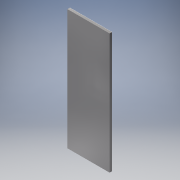
# Autodesk Inventor part: Etichetta
Saved by Autodesk Inventor 2016 (Build 200138000, 138)
## iProperties
Created: 2016-09-10
Part Number: Etichetta
Material: Generic
Document SubType Name: Modeling
Designer: Muhammad
Density: 1 g/cm^3
Appearance: Knurled 45
Author: Muhammad
Autodesk Inventor part; units mm, degrees
(part 1 of 2)
ref_plane "YZ Plane" through (0, 0, 0) normal (1, 0, 0) x (0, 1, 0)
ref_plane "XZ Plane" through (0, 0, 0) normal (0, 1, 0) x (-1, 0, 0)
ref_plane "XY Plane" through (0, 0, 0) normal (0, 0, 1) x (1, 0, 0)
sketch "Sketch1" plane through (0, 0, 0) normal (0, 1, 0) x (-1, 0, 0)
  line L0 (14, 40) -> (-14, 40)
  line L1 (-14, 40) -> (-14, -40)
  line L2 (-14, -40) -> (14, -40)
  line L3 (14, -40) -> (14, 40)
  line L4 (14, 40) -> (-14, -40) construction
  line L5 (-14, 40) -> (14, -40) construction
  point P0 (0, 0)
  dimension "d0" = 28
  dimension "d1" = 80
  constraints: 12 end point, 2 midpoint, 2 parallel, 1 horizontal, 1 perpendicular
  measures "d0" distance of L2.end L1.end
  measures "d1" distance of L1.end L0.end
extrude "Extrusion1" add sketch "Sketch1" along normal blind 2
fillet "Fillet1" radius 0.5 4 edges at (-14, 2, 0) (0, 2, 40) (14, 2, 0) (0, 2, -40)
sketch "Sketch3" plane through (0, 2, 0) normal (0, 1, 0) x (1, 0, 0)
  line L0 (-11.1237, -27.6216) -> (-11.1237, 26.8213) construction
  line L1 (-11.1237, 26.8213) -> (10.7875, 26.8213) construction
  line L2 (10.7875, 26.8213) -> (10.7875, -27.6216) construction
  line L3 (10.7875, -27.6216) -> (-11.1237, -27.6216) construction
  line L4 (-14, 40) -> (-14, -40) construction
  line L5 (-14, 0) -> (0, 0) construction
  spline S0 degree 2 poles (-8.5426, -15.8821) (-8.2817, -15.8821) (-7.8818, -16.0806) (-7.7513, -16.2451) knots 0 0 0 1 2 2 2
  spline S1 degree 2 poles (-7.7513, -16.2451) (-7.5982, -16.4437) (-7.4677, -16.8947) (-7.4677, -17.252) knots 0 0 0 1 2 2 2
  line L6 (-7.4677, -17.252) -> (-7.4677, -18.2561)
  line L7 (-7.4677, -18.2561) -> (-10.9677, -18.2561)
  line L8 (-10.9677, -18.2561) -> (-10.9677, -17.3286)
  spline S2 degree 2 poles (-10.9677, -17.3286) (-10.9677, -16.9542) (-10.9195, -16.5798) (-10.8259, -16.4097) knots 0 0 0 1 2 2 2
  spline S3 degree 2 poles (-10.8259, -16.4097) (-10.7266, -16.2196) (-10.4004, -16.0466) (-10.1792, -16.0466) knots 0 0 0 1 2 2 2
  spline S4 degree 2 poles (-10.1792, -16.0466) (-9.9324, -16.0466) (-9.541, -16.3075) (-9.4304, -16.5373) knots 0 0 0 1 2 2 2
  line L9 (-9.4304, -16.5373) -> (-9.4134, -16.5373)
  spline S5 degree 2 poles (-9.4134, -16.5373) (-9.3283, -16.2253) (-8.8773, -15.8821) (-8.5426, -15.8821) knots 0 0 0 1 2 2 2
  spline S6 degree 2 poles (-8.5228, -16.3671) (-8.7213, -16.3671) (-8.9766, -16.4806) (-9.0674, -16.6507) knots 0 0 0 1 2 2 2
  spline S7 degree 2 poles (-9.0674, -16.6507) (-9.1241, -16.7614) (-9.1581, -17.0223) (-9.1581, -17.2634) knots 0 0 0 1 2 2 2
  line L10 (-9.1581, -17.2634) -> (-9.1581, -17.7909)
  line L11 (-9.1581, -17.7909) -> (-7.8648, -17.7909)
  line L12 (-7.8648, -17.7909) -> (-7.8648, -17.4137)
  spline S8 degree 2 poles (-7.8648, -17.4137) (-7.8648, -17.1074) (-7.9215, -16.7557) (-8.0123, -16.6195) knots 0 0 0 1 2 2 2
  spline S9 degree 2 poles (-8.0123, -16.6195) (-8.1059, -16.4891) (-8.3384, -16.3671) (-8.5228, -16.3671) knots 0 0 0 1 2 2 2
  spline S10 degree 2 poles (-10.114, -16.5316) (-10.2388, -16.5316) (-10.426, -16.6167) (-10.4798, -16.7103) knots 0 0 0 1 2 2 2
  spline S11 degree 2 poles (-10.4798, -16.7103) (-10.5422, -16.8238) (-10.5706, -17.0989) (-10.5706, -17.3456) knots 0 0 0 1 2 2 2
  line L13 (-10.5706, -17.3456) -> (-10.5706, -17.7909)
  line L14 (-10.5706, -17.7909) -> (-9.5467, -17.7909)
  line L15 (-9.5467, -17.7909) -> (-9.5467, -17.2634)
  spline S12 degree 2 poles (-9.5467, -17.2634) (-9.5467, -17.045) (-9.5921, -16.8379) (-9.663, -16.7273) knots 0 0 0 1 2 2 2
  spline S13 degree 2 poles (-9.663, -16.7273) (-9.7311, -16.6195) (-9.9495, -16.5316) (-10.114, -16.5316) knots 0 0 0 1 2 2 2
  spline S14 degree 2 poles (-7.4081, -14.3136) (-7.4081, -14.9433) (-8.1144, -15.6353) (-8.7667, -15.6353) knots 0 0 0 1 2 2 2
  spline S15 degree 2 poles (-8.7667, -15.6353) (-9.4077, -15.6353) (-10.1678, -14.9631) (-10.1678, -14.4214) knots 0 0 0 1 2 2 2
  spline S16 degree 2 poles (-10.1678, -14.4214) (-10.1678, -14.1775) (-10.026, -13.8003) (-9.8757, -13.6613) knots 0 0 0 1 2 2 2
  spline S17 degree 2 poles (-9.8757, -13.6613) (-9.7254, -13.5195) (-9.2914, -13.3691) (-8.9766, -13.3691) knots 0 0 0 1 2 2 2
  line L16 (-8.9766, -13.3691) -> (-8.7355, -13.3691)
  line L17 (-8.7355, -13.3691) -> (-8.7355, -15.1872)
  spline S18 degree 2 poles (-8.7355, -15.1872) (-8.2789, -15.1872) (-7.7939, -14.7277) (-7.7939, -14.3193) knots 0 0 0 1 2 2 2
  spline S19 degree 2 poles (-7.7939, -14.3193) (-7.7939, -14.1746) (-7.8591, -13.8939) (-7.9102, -13.7804) knots 0 0 0 1 2 2 2
  spline S20 degree 2 poles (-7.9102, -13.7804) (-7.9669, -13.6613) (-8.0661, -13.4968) (-8.1115, -13.4429) knots 0 0 0 1 2 2 2
  line L18 (-8.1115, -13.4429) -> (-8.1115, -13.4174)
  line L19 (-8.1115, -13.4174) -> (-7.6294, -13.4174)
  spline S21 degree 2 poles (-7.6294, -13.4174) (-7.5982, -13.4939) (-7.5074, -13.7265) (-7.4819, -13.8173) knots 0 0 0 1 2 2 2
  spline S22 degree 2 poles (-7.4819, -13.8173) (-7.445, -13.9449) (-7.4081, -14.1548) (-7.4081, -14.3136) knots 0 0 0 1 2 2 2
  spline S23 degree 2 poles (-9.073, -13.8003) (-9.2517, -13.8059) (-9.5127, -13.8797) (-9.6006, -13.9506) knots 0 0 0 1 2 2 2
  spline S24 degree 2 poles (-9.6006, -13.9506) (-9.6999, -14.0272) (-9.8048, -14.2682) (-9.8048, -14.4469) knots 0 0 0 1 2 2 2
  spline S25 degree 2 poles (-9.8048, -14.4469) (-9.8048, -14.6228) (-9.6999, -14.8695) (-9.5978, -14.9716) knots 0 0 0 1 2 2 2
  spline S26 degree 2 poles (-9.5978, -14.9716) (-9.4928, -15.0709) (-9.2404, -15.173) (-9.073, -15.1872) knots 0 0 0 1 2 2 2
  line L20 (-9.073, -15.1872) -> (-9.073, -13.8003)
  line L21 (-9.6204, -11.5284) -> (-9.6204, -11.5511)
  spline S27 degree 2 poles (-9.6204, -11.5511) (-9.6346, -11.6021) (-9.6403, -11.7127) (-9.6403, -11.7893) knots 0 0 0 1 2 2 2
  spline S28 degree 2 poles (-9.6403, -11.7893) (-9.6403, -11.968) (-9.4843, -12.3197) (-9.3311, -12.4785) knots 0 0 0 1 2 2 2
  line L22 (-9.3311, -12.4785) -> (-7.4677, -12.4785)
  line L23 (-7.4677, -12.4785) -> (-7.4677, -12.921)
  line L24 (-7.4677, -12.921) -> (-10.0941, -12.921)
  line L25 (-10.0941, -12.921) -> (-10.0941, -12.4785)
  line L26 (-10.0941, -12.4785) -> (-9.7027, -12.4785)
  spline S29 degree 2 poles (-9.7027, -12.4785) (-9.9183, -12.2375) (-10.0941, -11.8772) (-10.0941, -11.7071) knots 0 0 0 1 2 2 2
  spline S30 degree 2 poles (-10.0941, -11.7071) (-10.0941, -11.639) (-10.0884, -11.5709) (-10.0799, -11.5284) knots 0 0 0 1 2 2 2
  line L27 (-10.0799, -11.5284) -> (-9.6204, -11.5284)
  line L28 (-7.4677, -9.1232) -> (-7.4677, -9.5657)
  line L29 (-7.4677, -9.5657) -> (-8.9653, -9.5657)
  spline S31 degree 2 poles (-8.9653, -9.5657) (-9.1468, -9.5657) (-9.4588, -9.5997) (-9.5524, -9.6507) knots 0 0 0 1 2 2 2
  spline S32 degree 2 poles (-9.5524, -9.6507) (-9.6516, -9.7046) (-9.7481, -9.8975) (-9.7481, -10.062) knots 0 0 0 1 2 2 2
  spline S33 degree 2 poles (-9.7481, -10.062) (-9.7481, -10.2265) (-9.5722, -10.5754) (-9.4304, -10.7427) knots 0 0 0 1 2 2 2
  line L30 (-9.4304, -10.7427) -> (-7.4677, -10.7427)
  line L31 (-7.4677, -10.7427) -> (-7.4677, -11.1852)
  line L32 (-7.4677, -11.1852) -> (-10.0941, -11.1852)
  line L33 (-10.0941, -11.1852) -> (-10.0941, -10.7427)
  line L34 (-10.0941, -10.7427) -> (-9.802, -10.7427)
  spline S34 degree 2 poles (-9.802, -10.7427) (-9.9807, -10.5442) (-10.1678, -10.1613) (-10.1678, -9.9457) knots 0 0 0 1 2 2 2
  spline S35 degree 2 poles (-10.1678, -9.9457) (-10.1678, -9.56) (-9.6573, -9.1232) (-9.1723, -9.1232) knots 0 0 0 1 2 2 2
  line L35 (-9.1723, -9.1232) -> (-7.4677, -9.1232)
  spline S36 degree 2 poles (-7.7456, -7.0385) (-7.7059, -7.0924) (-7.5641, -7.2739) (-7.5216, -7.359) knots 0 0 0 1 2 2 2
  spline S37 degree 2 poles (-7.5216, -7.359) (-7.4592, -7.4753) (-7.3939, -7.6937) (-7.3939, -7.8922) knots 0 0 0 1 2 2 2
  spline S38 degree 2 poles (-7.3939, -7.8922) (-7.3939, -8.0539) (-7.5159, -8.346) (-7.6265, -8.4567) knots 0 0 0 1 2 2 2
  spline S39 degree 2 poles (-7.6265, -8.4567) (-7.7343, -8.5616) (-8.052, -8.6892) (-8.2278, -8.6892) knots 0 0 0 1 2 2 2
  spline S40 degree 2 poles (-8.2278, -8.6892) (-8.5001, -8.6892) (-8.8858, -8.4595) (-8.9965, -8.2099) knots 0 0 0 1 2 2 2
  spline S41 degree 2 poles (-8.9965, -8.2099) (-9.0986, -7.9887) (-9.1751, -7.3874) (-9.195, -7.0385) knots 0 0 0 1 2 2 2
  line L36 (-9.195, -7.0385) -> (-9.2801, -7.0385)
  spline S42 degree 2 poles (-9.2801, -7.0385) (-9.4332, -7.0385) (-9.6233, -7.1321) (-9.6772, -7.2172) knots 0 0 0 1 2 2 2
  spline S43 degree 2 poles (-9.6772, -7.2172) (-9.7311, -7.3023) (-9.7651, -7.5462) (-9.7651, -7.6767) knots 0 0 0 1 2 2 2
  spline S44 degree 2 poles (-9.7651, -7.6767) (-9.7651, -7.8298) (-9.6743, -8.2439) (-9.5864, -8.451) knots 0 0 0 1 2 2 2
  line L37 (-9.5864, -8.451) -> (-9.5864, -8.4765)
  line L38 (-9.5864, -8.4765) -> (-10.0374, -8.4765)
  spline S45 degree 2 poles (-10.0374, -8.4765) (-10.0714, -8.3546) (-10.1565, -7.8979) (-10.1565, -7.6738) knots 0 0 0 1 2 2 2
  spline S46 degree 2 poles (-10.1565, -7.6738) (-10.1565, -7.4016) (-10.0714, -7.03) (-9.9608, -6.8825) knots 0 0 0 1 2 2 2
  spline S47 degree 2 poles (-9.9608, -6.8825) (-9.853, -6.7379) (-9.5098, -6.596) (-9.2631, -6.596) knots 0 0 0 1 2 2 2
  line L39 (-9.2631, -6.596) -> (-7.4677, -6.596)
  line L40 (-7.4677, -6.596) -> (-7.4677, -7.0385)
  line L41 (-7.4677, -7.0385) -> (-7.7456, -7.0385)
  line L42 (-8.1144, -7.0385) -> (-8.8433, -7.0385)
  spline S48 degree 2 poles (-8.8433, -7.0385) (-8.8291, -7.1973) (-8.7809, -7.6767) (-8.7355, -7.827) knots 0 0 0 1 2 2 2
  spline S49 degree 2 poles (-8.7355, -7.827) (-8.6816, -8.0028) (-8.4576, -8.2326) (-8.259, -8.2326) knots 0 0 0 1 2 2 2
  spline S50 degree 2 poles (-8.259, -8.2326) (-8.0321, -8.2326) (-7.8024, -7.9773) (-7.8024, -7.7334) knots 0 0 0 1 2 2 2
  spline S51 degree 2 poles (-7.8024, -7.7334) (-7.8024, -7.5263) (-7.9811, -7.186) (-8.1144, -7.0385) knots 0 0 0 1 2 2 2
  line L43 (-10.0941, -3.9129) -> (-6.5005, -5.3254)
  line L44 (-6.5005, -5.3254) -> (-6.5005, -5.799)
  line L45 (-6.5005, -5.799) -> (-7.5953, -5.3282)
  line L46 (-7.5953, -5.3282) -> (-10.0941, -6.2812)
  line L47 (-10.0941, -6.2812) -> (-10.0941, -5.8047)
  line L48 (-10.0941, -5.8047) -> (-8.1484, -5.0871)
  line L49 (-8.1484, -5.0871) -> (-10.0941, -4.3724)
  line L50 (-10.0941, -4.3724) -> (-10.0941, -3.9129)
  spline S52 degree 2 poles (-7.4053, -2.8691) (-7.4053, -3.1329) (-7.5471, -3.5896) (-7.6265, -3.7399) knots 0 0 0 1 2 2 2
  line L51 (-7.6265, -3.7399) -> (-8.1229, -3.7399)
  line L52 (-8.1229, -3.7399) -> (-8.1229, -3.7172)
  spline S53 degree 2 poles (-8.1229, -3.7172) (-8.0775, -3.6605) (-7.9697, -3.5073) (-7.9102, -3.3797) knots 0 0 0 1 2 2 2
  spline S54 degree 2 poles (-7.9102, -3.3797) (-7.8563, -3.2691) (-7.7768, -2.9968) (-7.7768, -2.8521) knots 0 0 0 1 2 2 2
  spline S55 degree 2 poles (-7.7768, -2.8521) (-7.7768, -2.7472) (-7.8251, -2.5061) (-7.8648, -2.4494) knots 0 0 0 1 2 2 2
  spline S56 degree 2 poles (-7.8648, -2.4494) (-7.9187, -2.3671) (-8.0406, -2.2934) (-8.1654, -2.2934) knots 0 0 0 1 2 2 2
  spline S57 degree 2 poles (-8.1654, -2.2934) (-8.3214, -2.2934) (-8.4831, -2.4635) (-8.537, -2.6819) knots 0 0 0 1 2 2 2
  spline S58 degree 2 poles (-8.537, -2.6819) (-8.5568, -2.767) (-8.6136, -3.0393) (-8.6448, -3.1556) knots 0 0 0 1 2 2 2
  spline S59 degree 2 poles (-8.6448, -3.1556) (-8.7327, -3.4563) (-9.0957, -3.7285) (-9.3538, -3.7285) knots 0 0 0 1 2 2 2
  spline S60 degree 2 poles (-9.3538, -3.7285) (-9.7112, -3.7285) (-10.1565, -3.1925) (-10.1565, -2.75) knots 0 0 0 1 2 2 2
  spline S61 degree 2 poles (-10.1565, -2.75) (-10.1565, -2.5316) (-10.0487, -2.0892) (-9.9665, -1.9388) knots 0 0 0 1 2 2 2
  line L53 (-9.9665, -1.9388) -> (-9.4928, -1.9388)
  line L54 (-9.4928, -1.9388) -> (-9.4928, -1.9615)
  spline S62 degree 2 poles (-9.4928, -1.9615) (-9.629, -2.1317) (-9.7849, -2.5458) (-9.7849, -2.7585) knots 0 0 0 1 2 2 2
  spline S63 degree 2 poles (-9.7849, -2.7585) (-9.7849, -2.9769) (-9.6006, -3.2776) (-9.4162, -3.2776) knots 0 0 0 1 2 2 2
  spline S64 degree 2 poles (-9.4162, -3.2776) (-9.2489, -3.2776) (-9.0872, -3.0989) (-9.0362, -2.9003) knots 0 0 0 1 2 2 2
  spline S65 degree 2 poles (-9.0362, -2.9003) (-9.0106, -2.8039) (-8.9596, -2.56) (-8.9284, -2.4267) knots 0 0 0 1 2 2 2
  spline S66 degree 2 poles (-8.9284, -2.4267) (-8.8546, -2.1374) (-8.5171, -1.8424) (-8.225, -1.8424) knots 0 0 0 1 2 2 2
  spline S67 degree 2 poles (-8.225, -1.8424) (-8.0548, -1.8424) (-7.7542, -1.9757) (-7.6435, -2.1062) knots 0 0 0 1 2 2 2
  spline S68 degree 2 poles (-7.6435, -2.1062) (-7.5272, -2.2452) (-7.4053, -2.5997) (-7.4053, -2.8691) knots 0 0 0 1 2 2 2
  line L55 (-11.1237, -0.983) -> (-9.7623, -1.0851)
  line L56 (-9.7623, -1.0851) -> (-9.7623, -1.4028)
  line L57 (-9.7623, -1.4028) -> (-11.1237, -1.5049)
  line L58 (-11.1237, -1.5049) -> (-11.1237, -0.983)
  spline S69 degree 2 poles (-7.4053, 0.2933) (-7.4053, 0.0296) (-7.5471, -0.4271) (-7.6265, -0.5774) knots 0 0 0 1 2 2 2
  line L59 (-7.6265, -0.5774) -> (-8.1229, -0.5774)
  line L60 (-8.1229, -0.5774) -> (-8.1229, -0.5547)
  spline S70 degree 2 poles (-8.1229, -0.5547) (-8.0775, -0.498) (-7.9697, -0.3448) (-7.9102, -0.2172) knots 0 0 0 1 2 2 2
  spline S71 degree 2 poles (-7.9102, -0.2172) (-7.8563, -0.1066) (-7.7768, 0.1657) (-7.7768, 0.3104) knots 0 0 0 1 2 2 2
  spline S72 degree 2 poles (-7.7768, 0.3104) (-7.7768, 0.4153) (-7.8251, 0.6564) (-7.8648, 0.7131) knots 0 0 0 1 2 2 2
  spline S73 degree 2 poles (-7.8648, 0.7131) (-7.9187, 0.7954) (-8.0406, 0.8691) (-8.1654, 0.8691) knots 0 0 0 1 2 2 2
  spline S74 degree 2 poles (-8.1654, 0.8691) (-8.3214, 0.8691) (-8.4831, 0.6989) (-8.537, 0.4805) knots 0 0 0 1 2 2 2
  spline S75 degree 2 poles (-8.537, 0.4805) (-8.5568, 0.3954) (-8.6136, 0.1232) (-8.6448, 0.0069) knots 0 0 0 1 2 2 2
  spline S76 degree 2 poles (-8.6448, 0.0069) (-8.7327, -0.2938) (-9.0957, -0.5661) (-9.3538, -0.5661) knots 0 0 0 1 2 2 2
  spline S77 degree 2 poles (-9.3538, -0.5661) (-9.7112, -0.5661) (-10.1565, -0.03) (-10.1565, 0.4125) knots 0 0 0 1 2 2 2
  spline S78 degree 2 poles (-10.1565, 0.4125) (-10.1565, 0.6309) (-10.0487, 1.0733) (-9.9665, 1.2237) knots 0 0 0 1 2 2 2
  line L61 (-9.9665, 1.2237) -> (-9.4928, 1.2237)
  line L62 (-9.4928, 1.2237) -> (-9.4928, 1.201)
  spline S79 degree 2 poles (-9.4928, 1.201) (-9.629, 1.0308) (-9.7849, 0.6167) (-9.7849, 0.404) knots 0 0 0 1 2 2 2
  spline S80 degree 2 poles (-9.7849, 0.404) (-9.7849, 0.1856) (-9.6006, -0.1151) (-9.4162, -0.1151) knots 0 0 0 1 2 2 2
  spline S81 degree 2 poles (-9.4162, -0.1151) (-9.2489, -0.1151) (-9.0872, 0.0636) (-9.0362, 0.2621) knots 0 0 0 1 2 2 2
  spline S82 degree 2 poles (-9.0362, 0.2621) (-9.0106, 0.3586) (-8.9596, 0.6025) (-8.9284, 0.7358) knots 0 0 0 1 2 2 2
  spline S83 degree 2 poles (-8.9284, 0.7358) (-8.8546, 1.0251) (-8.5171, 1.3201) (-8.225, 1.3201) knots 0 0 0 1 2 2 2
  spline S84 degree 2 poles (-8.225, 1.3201) (-8.0548, 1.3201) (-7.7542, 1.1868) (-7.6435, 1.0563) knots 0 0 0 1 2 2 2
  spline S85 degree 2 poles (-7.6435, 1.0563) (-7.5272, 0.9173) (-7.4053, 0.5628) (-7.4053, 0.2933) knots 0 0 0 1 2 2 2
  spline S86 degree 2 poles (-7.4053, 4.2443) (-7.4053, 3.8643) (-7.5641, 3.331) (-7.6776, 3.0956) knots 0 0 0 1 2 2 2
  line L63 (-7.6776, 3.0956) -> (-8.2619, 3.0956)
  line L64 (-8.2619, 3.0956) -> (-8.2619, 3.1296)
  spline S87 degree 2 poles (-8.2619, 3.1296) (-8.0463, 3.3594) (-7.808, 3.9408) (-7.808, 4.2103) knots 0 0 0 1 2 2 2
  spline S88 degree 2 poles (-7.808, 4.2103) (-7.808, 4.596) (-8.1285, 4.9903) (-8.3923, 4.9903) knots 0 0 0 1 2 2 2
  spline S89 degree 2 poles (-8.3923, 4.9903) (-8.6022, 4.9903) (-8.8631, 4.7832) (-8.9284, 4.5591) knots 0 0 0 1 2 2 2
  spline S90 degree 2 poles (-8.9284, 4.5591) (-8.9738, 4.3975) (-9.0362, 4.128) (-9.0872, 3.9266) knots 0 0 0 1 2 2 2
  spline S91 degree 2 poles (-9.0872, 3.9266) (-9.1354, 3.7451) (-9.2801, 3.4587) (-9.3964, 3.348) knots 0 0 0 1 2 2 2
  spline S92 degree 2 poles (-9.3964, 3.348) (-9.5127, 3.2403) (-9.8247, 3.1211) (-10.0289, 3.1211) knots 0 0 0 1 2 2 2
  spline S93 degree 2 poles (-10.0289, 3.1211) (-10.4543, 3.1211) (-11.0301, 3.7848) (-11.0301, 4.2982) knots 0 0 0 1 2 2 2
  spline S94 degree 2 poles (-11.0301, 4.2982) (-11.0301, 4.5932) (-10.9138, 5.1151) (-10.8032, 5.3391) knots 0 0 0 1 2 2 2
  line L65 (-10.8032, 5.3391) -> (-10.2473, 5.3391)
  line L66 (-10.2473, 5.3391) -> (-10.2473, 5.3051)
  spline S95 degree 2 poles (-10.2473, 5.3051) (-10.4004, 5.1378) (-10.6273, 4.6159) (-10.6273, 4.3294) knots 0 0 0 1 2 2 2
  spline S96 degree 2 poles (-10.6273, 4.3294) (-10.6273, 4.0061) (-10.3238, 3.6061) (-10.0771, 3.6061) knots 0 0 0 1 2 2 2
  spline S97 degree 2 poles (-10.0771, 3.6061) (-9.8559, 3.6061) (-9.5921, 3.8416) (-9.5325, 4.0628) knots 0 0 0 1 2 2 2
  spline S98 degree 2 poles (-9.5325, 4.0628) (-9.4928, 4.2103) (-9.3907, 4.6386) (-9.3482, 4.7804) knots 0 0 0 1 2 2 2
  spline S99 degree 2 poles (-9.3482, 4.7804) (-9.2375, 5.1406) (-8.7922, 5.4753) (-8.4661, 5.4753) knots 0 0 0 1 2 2 2
  spline S100 degree 2 poles (-8.4661, 5.4753) (-8.259, 5.4753) (-7.8619, 5.3079) (-7.723, 5.1576) knots 0 0 0 1 2 2 2
  spline S101 degree 2 poles (-7.723, 5.1576) (-7.5698, 4.9903) (-7.4053, 4.5648) (-7.4053, 4.2443) knots 0 0 0 1 2 2 2
  spline S102 degree 2 poles (-7.4166, 6.7091) (-7.4166, 6.3489) (-7.8279, 5.9433) (-8.2732, 5.9433) knots 0 0 0 1 2 2 2
  line L67 (-8.2732, 5.9433) -> (-9.7282, 5.9433)
  line L68 (-9.7282, 5.9433) -> (-9.7282, 5.6454)
  line L69 (-9.7282, 5.6454) -> (-10.0941, 5.6454)
  line L70 (-10.0941, 5.6454) -> (-10.0941, 5.9433)
  line L71 (-10.0941, 5.9433) -> (-10.8486, 5.9433)
  line L72 (-10.8486, 5.9433) -> (-10.8486, 6.3857)
  line L73 (-10.8486, 6.3857) -> (-10.0941, 6.3857)
  line L74 (-10.0941, 6.3857) -> (-10.0941, 7.1997)
  line L75 (-10.0941, 7.1997) -> (-9.7282, 7.1997)
  line L76 (-9.7282, 7.1997) -> (-9.7282, 6.3857)
  line L77 (-9.7282, 6.3857) -> (-8.4774, 6.3857)
  spline S103 degree 2 poles (-8.4774, 6.3857) (-8.2789, 6.3857) (-8.0605, 6.3999) (-7.9669, 6.4481) knots 0 0 0 1 2 2 2
  spline S104 degree 2 poles (-7.9669, 6.4481) (-7.8846, 6.4878) (-7.8024, 6.6665) (-7.8024, 6.8197) knots 0 0 0 1 2 2 2
  spline S105 degree 2 poles (-7.8024, 6.8197) (-7.8024, 6.9275) (-7.8676, 7.1288) (-7.8875, 7.1742) knots 0 0 0 1 2 2 2
  line L78 (-7.8875, 7.1742) -> (-7.8875, 7.1997)
  line L79 (-7.8875, 7.1997) -> (-7.4904, 7.1997)
  spline S106 degree 2 poles (-7.4904, 7.1997) (-7.4563, 7.0749) (-7.4166, 6.8197) (-7.4166, 6.7091) knots 0 0 0 1 2 2 2
  spline S107 degree 2 poles (-7.4081, 8.6661) (-7.4081, 8.0365) (-8.1144, 7.3444) (-8.7667, 7.3444) knots 0 0 0 1 2 2 2
  spline S108 degree 2 poles (-8.7667, 7.3444) (-9.4077, 7.3444) (-10.1678, 8.0166) (-10.1678, 8.5583) knots 0 0 0 1 2 2 2
  spline S109 degree 2 poles (-10.1678, 8.5583) (-10.1678, 8.8023) (-10.026, 9.1795) (-9.8757, 9.3185) knots 0 0 0 1 2 2 2
  spline S110 degree 2 poles (-9.8757, 9.3185) (-9.7254, 9.4603) (-9.2914, 9.6106) (-8.9766, 9.6106) knots 0 0 0 1 2 2 2
  line L80 (-8.9766, 9.6106) -> (-8.7355, 9.6106)
  line L81 (-8.7355, 9.6106) -> (-8.7355, 7.7925)
  spline S111 degree 2 poles (-8.7355, 7.7925) (-8.2789, 7.7925) (-7.7939, 8.252) (-7.7939, 8.6604) knots 0 0 0 1 2 2 2
  spline S112 degree 2 poles (-7.7939, 8.6604) (-7.7939, 8.8051) (-7.8591, 9.0859) (-7.9102, 9.1993) knots 0 0 0 1 2 2 2
  spline S113 degree 2 poles (-7.9102, 9.1993) (-7.9669, 9.3185) (-8.0661, 9.483) (-8.1115, 9.5369) knots 0 0 0 1 2 2 2
  line L82 (-8.1115, 9.5369) -> (-8.1115, 9.5624)
  line L83 (-8.1115, 9.5624) -> (-7.6294, 9.5624)
  spline S114 degree 2 poles (-7.6294, 9.5624) (-7.5982, 9.4858) (-7.5074, 9.2532) (-7.4819, 9.1625) knots 0 0 0 1 2 2 2
  spline S115 degree 2 poles (-7.4819, 9.1625) (-7.445, 9.0348) (-7.4081, 8.8249) (-7.4081, 8.6661) knots 0 0 0 1 2 2 2
  spline S116 degree 2 poles (-9.073, 9.1795) (-9.2517, 9.1738) (-9.5127, 9.1001) (-9.6006, 9.0292) knots 0 0 0 1 2 2 2
  spline S117 degree 2 poles (-9.6006, 9.0292) (-9.6999, 8.9526) (-9.8048, 8.7115) (-9.8048, 8.5328) knots 0 0 0 1 2 2 2
  spline S118 degree 2 poles (-9.8048, 8.5328) (-9.8048, 8.357) (-9.6999, 8.1102) (-9.5978, 8.0081) knots 0 0 0 1 2 2 2
  spline S119 degree 2 poles (-9.5978, 8.0081) (-9.4928, 7.9088) (-9.2404, 7.8067) (-9.073, 7.7925) knots 0 0 0 1 2 2 2
  line L84 (-9.073, 7.7925) -> (-9.073, 9.1795)
  spline S120 degree 2 poles (-7.7456, 11.5223) (-7.7059, 11.4684) (-7.5641, 11.2869) (-7.5216, 11.2018) knots 0 0 0 1 2 2 2
  spline S121 degree 2 poles (-7.5216, 11.2018) (-7.4592, 11.0855) (-7.3939, 10.8671) (-7.3939, 10.6685) knots 0 0 0 1 2 2 2
  spline S122 degree 2 poles (-7.3939, 10.6685) (-7.3939, 10.5069) (-7.5159, 10.2147) (-7.6265, 10.1041) knots 0 0 0 1 2 2 2
  spline S123 degree 2 poles (-7.6265, 10.1041) (-7.7343, 9.9992) (-8.052, 9.8715) (-8.2278, 9.8715) knots 0 0 0 1 2 2 2
  spline S124 degree 2 poles (-8.2278, 9.8715) (-8.5001, 9.8715) (-8.8858, 10.1013) (-8.9965, 10.3509) knots 0 0 0 1 2 2 2
  spline S125 degree 2 poles (-8.9965, 10.3509) (-9.0986, 10.5721) (-9.1751, 11.1734) (-9.195, 11.5223) knots 0 0 0 1 2 2 2
  line L85 (-9.195, 11.5223) -> (-9.2801, 11.5223)
  spline S126 degree 2 poles (-9.2801, 11.5223) (-9.4332, 11.5223) (-9.6233, 11.4287) (-9.6772, 11.3436) knots 0 0 0 1 2 2 2
  spline S127 degree 2 poles (-9.6772, 11.3436) (-9.7311, 11.2585) (-9.7651, 11.0146) (-9.7651, 10.8841) knots 0 0 0 1 2 2 2
  spline S128 degree 2 poles (-9.7651, 10.8841) (-9.7651, 10.7309) (-9.6743, 10.3168) (-9.5864, 10.1098) knots 0 0 0 1 2 2 2
  line L86 (-9.5864, 10.1098) -> (-9.5864, 10.0843)
  line L87 (-9.5864, 10.0843) -> (-10.0374, 10.0843)
  spline S129 degree 2 poles (-10.0374, 10.0843) (-10.0714, 10.2062) (-10.1565, 10.6629) (-10.1565, 10.8869) knots 0 0 0 1 2 2 2
  spline S130 degree 2 poles (-10.1565, 10.8869) (-10.1565, 11.1592) (-10.0714, 11.5308) (-9.9608, 11.6783) knots 0 0 0 1 2 2 2
  spline S131 degree 2 poles (-9.9608, 11.6783) (-9.853, 11.8229) (-9.5098, 11.9647) (-9.2631, 11.9647) knots 0 0 0 1 2 2 2
  line L88 (-9.2631, 11.9647) -> (-7.4677, 11.9647)
  line L89 (-7.4677, 11.9647) -> (-7.4677, 11.5223)
  line L90 (-7.4677, 11.5223) -> (-7.7456, 11.5223)
  line L91 (-8.1144, 11.5223) -> (-8.8433, 11.5223)
  spline S132 degree 2 poles (-8.8433, 11.5223) (-8.8291, 11.3634) (-8.7809, 10.8841) (-8.7355, 10.7338) knots 0 0 0 1 2 2 2
  spline S133 degree 2 poles (-8.7355, 10.7338) (-8.6816, 10.5579) (-8.4576, 10.3282) (-8.259, 10.3282) knots 0 0 0 1 2 2 2
  spline S134 degree 2 poles (-8.259, 10.3282) (-8.0321, 10.3282) (-7.8024, 10.5835) (-7.8024, 10.8274) knots 0 0 0 1 2 2 2
  spline S135 degree 2 poles (-7.8024, 10.8274) (-7.8024, 11.0344) (-7.9811, 11.3748) (-8.1144, 11.5223) knots 0 0 0 1 2 2 2
  line L92 (-7.4677, 15.564) -> (-8.9879, 15.564)
  spline S136 degree 2 poles (-8.9879, 15.564) (-9.1695, 15.564) (-9.4786, 15.5356) (-9.5637, 15.4903) knots 0 0 0 1 2 2 2
  spline S137 degree 2 poles (-9.5637, 15.4903) (-9.6573, 15.4449) (-9.7481, 15.2719) (-9.7481, 15.1215) knots 0 0 0 1 2 2 2
  spline S138 degree 2 poles (-9.7481, 15.1215) (-9.7481, 14.9854) (-9.5807, 14.6734) (-9.4219, 14.5089) knots 0 0 0 1 2 2 2
  spline S139 degree 2 poles (-9.4219, 14.5089) (-9.3822, 14.5117) (-9.2716, 14.5174) (-9.1978, 14.5174) knots 0 0 0 1 2 2 2
  line L93 (-9.1978, 14.5174) -> (-7.4677, 14.5174)
  line L94 (-7.4677, 14.5174) -> (-7.4677, 14.0749)
  line L95 (-7.4677, 14.0749) -> (-8.9879, 14.0749)
  spline S140 degree 2 poles (-8.9879, 14.0749) (-9.1695, 14.0749) (-9.4786, 14.0466) (-9.5637, 14.0012) knots 0 0 0 1 2 2 2
  spline S141 degree 2 poles (-9.5637, 14.0012) (-9.6573, 13.9558) (-9.7481, 13.7828) (-9.7481, 13.6325) knots 0 0 0 1 2 2 2
  spline S142 degree 2 poles (-9.7481, 13.6325) (-9.7481, 13.4907) (-9.5694, 13.1758) (-9.4304, 13.0284) knots 0 0 0 1 2 2 2
  line L96 (-9.4304, 13.0284) -> (-7.4677, 13.0284)
  line L97 (-7.4677, 13.0284) -> (-7.4677, 12.5859)
  line L98 (-7.4677, 12.5859) -> (-10.0941, 12.5859)
  line L99 (-10.0941, 12.5859) -> (-10.0941, 13.0284)
  line L100 (-10.0941, 13.0284) -> (-9.8048, 13.0284)
  spline S143 degree 2 poles (-9.8048, 13.0284) (-9.9778, 13.2014) (-10.1678, 13.5417) (-10.1678, 13.7459) knots 0 0 0 1 2 2 2
  spline S144 degree 2 poles (-10.1678, 13.7459) (-10.1678, 13.9785) (-9.9551, 14.3387) (-9.714, 14.4323) knots 0 0 0 1 2 2 2
  spline S145 degree 2 poles (-9.714, 14.4323) (-9.9381, 14.6337) (-10.1678, 15.0138) (-10.1678, 15.235) knots 0 0 0 1 2 2 2
  spline S146 degree 2 poles (-10.1678, 15.235) (-10.1678, 15.4052) (-10.0629, 15.6831) (-9.9438, 15.7852) knots 0 0 0 1 2 2 2
  spline S147 degree 2 poles (-9.9438, 15.7852) (-9.8247, 15.8902) (-9.4673, 16.0065) (-9.1978, 16.0065) knots 0 0 0 1 2 2 2
  line L101 (-9.1978, 16.0065) -> (-7.4677, 16.0065)
  line L102 (-7.4677, 16.0065) -> (-7.4677, 15.564)
  line L103 (-1.705, -7.9773) -> (-5.205, -7.9773)
  line L104 (-5.205, -7.9773) -> (-5.205, -5.7877)
  line L105 (-5.205, -5.7877) -> (-4.7909, -5.7877)
  line L106 (-4.7909, -5.7877) -> (-4.7909, -7.5122)
  line L107 (-4.7909, -7.5122) -> (-3.8323, -7.5122)
  line L108 (-3.8323, -7.5122) -> (-3.8323, -5.904)
  line L109 (-3.8323, -5.904) -> (-3.4182, -5.904)
  line L110 (-3.4182, -5.904) -> (-3.4182, -7.5122)
  line L111 (-3.4182, -7.5122) -> (-2.1191, -7.5122)
  line L112 (-2.1191, -7.5122) -> (-2.1191, -5.7877)
  line L113 (-2.1191, -5.7877) -> (-1.705, -5.7877)
  line L114 (-1.705, -5.7877) -> (-1.705, -7.9773)
  line L115 (-1.705, -3.2492) -> (-1.705, -3.6917)
  line L116 (-1.705, -3.6917) -> (-3.2026, -3.6917)
  spline S148 degree 2 poles (-3.2026, -3.6917) (-3.3841, -3.6917) (-3.6961, -3.7257) (-3.7897, -3.7768) knots 0 0 0 1 2 2 2
  spline S149 degree 2 poles (-3.7897, -3.7768) (-3.889, -3.8306) (-3.9854, -4.0235) (-3.9854, -4.188) knots 0 0 0 1 2 2 2
  spline S150 degree 2 poles (-3.9854, -4.188) (-3.9854, -4.3525) (-3.8096, -4.7014) (-3.6678, -4.8687) knots 0 0 0 1 2 2 2
  line L117 (-3.6678, -4.8687) -> (-1.705, -4.8687)
  line L118 (-1.705, -4.8687) -> (-1.705, -5.3112)
  line L119 (-1.705, -5.3112) -> (-4.3314, -5.3112)
  line L120 (-4.3314, -5.3112) -> (-4.3314, -4.8687)
  line L121 (-4.3314, -4.8687) -> (-4.0393, -4.8687)
  spline S151 degree 2 poles (-4.0393, -4.8687) (-4.218, -4.6702) (-4.4052, -4.2873) (-4.4052, -4.0717) knots 0 0 0 1 2 2 2
  spline S152 degree 2 poles (-4.4052, -4.0717) (-4.4052, -3.686) (-3.8947, -3.2492) (-3.4096, -3.2492) knots 0 0 0 1 2 2 2
  line L122 (-3.4096, -3.2492) -> (-1.705, -3.2492)
  spline S153 degree 2 poles (-1.2853, -2.5345) (-1.2654, -2.4891) (-1.203, -2.3161) (-1.1775, -2.2054) knots 0 0 0 1 2 2 2
  spline S154 degree 2 poles (-1.1775, -2.2054) (-1.1463, -2.0835) (-1.1094, -1.8764) (-1.1094, -1.7545) knots 0 0 0 1 2 2 2
  spline S155 degree 2 poles (-1.1094, -1.7545) (-1.1094, -1.5503) (-1.2172, -1.2666) (-1.3136, -1.1872) knots 0 0 0 1 2 2 2
  spline S156 degree 2 poles (-1.3136, -1.1872) (-1.4101, -1.1106) (-1.6625, -1.0511) (-1.8242, -1.0511) knots 0 0 0 1 2 2 2
  line L123 (-1.8242, -1.0511) -> (-2.0539, -1.0511)
  spline S157 degree 2 poles (-2.0539, -1.0511) (-1.8979, -1.2298) (-1.7504, -1.5729) (-1.7504, -1.831) knots 0 0 0 1 2 2 2
  spline S158 degree 2 poles (-1.7504, -1.831) (-1.7504, -2.2792) (-2.4169, -2.8096) (-3.0438, -2.8096) knots 0 0 0 1 2 2 2
  spline S159 degree 2 poles (-3.0438, -2.8096) (-3.3699, -2.8096) (-3.8748, -2.6252) (-4.0535, -2.4721) knots 0 0 0 1 2 2 2
  spline S160 degree 2 poles (-4.0535, -2.4721) (-4.2208, -2.3246) (-4.4052, -1.919) (-4.4052, -1.7034) knots 0 0 0 1 2 2 2
  spline S161 degree 2 poles (-4.4052, -1.7034) (-4.4052, -1.4992) (-4.3088, -1.2014) (-4.2208, -1.0511) knots 0 0 0 1 2 2 2
  line L124 (-4.2208, -1.0511) -> (-4.3314, -1.0255)
  line L125 (-4.3314, -1.0255) -> (-4.3314, -0.6086)
  line L126 (-4.3314, -0.6086) -> (-2.0057, -0.6086)
  spline S162 degree 2 poles (-2.0057, -0.6086) (-1.3363, -0.6086) (-0.7123, -1.19) (-0.7123, -1.7885) knots 0 0 0 1 2 2 2
  spline S163 degree 2 poles (-0.7123, -1.7885) (-0.7123, -1.9814) (-0.7747, -2.3841) (-0.8258, -2.5571) knots 0 0 0 1 2 2 2
  line L127 (-0.8258, -2.5571) -> (-1.2853, -2.5571)
  line L128 (-1.2853, -2.5571) -> (-1.2853, -2.5345)
  line L129 (-2.4169, -1.0511) -> (-3.8606, -1.0511)
  spline S164 degree 2 poles (-3.8606, -1.0511) (-3.94, -1.2156) (-4.0081, -1.4935) (-4.0081, -1.6325) knots 0 0 0 1 2 2 2
  spline S165 degree 2 poles (-4.0081, -1.6325) (-4.0081, -1.9672) (-3.5146, -2.3529) (-3.0523, -2.3529) knots 0 0 0 1 2 2 2
  spline S166 degree 2 poles (-3.0523, -2.3529) (-2.6155, -2.3529) (-2.1588, -2.0608) (-2.1588, -1.7318) knots 0 0 0 1 2 2 2
  spline S167 degree 2 poles (-2.1588, -1.7318) (-2.1588, -1.5588) (-2.295, -1.1957) (-2.4169, -1.0511) knots 0 0 0 1 2 2 2
  line L130 (-1.705, 0.4834) -> (-1.705, 0.0409)
  line L131 (-1.705, 0.0409) -> (-4.3314, 0.0409)
  line L132 (-4.3314, 0.0409) -> (-4.3314, 0.4834)
  line L133 (-4.3314, 0.4834) -> (-1.705, 0.4834)
  line L134 (-4.7682, 0.5146) -> (-4.7682, 0.0125)
  line L135 (-4.7682, 0.0125) -> (-5.2277, 0.0125)
  line L136 (-5.2277, 0.0125) -> (-5.2277, 0.5146)
  line L137 (-5.2277, 0.5146) -> (-4.7682, 0.5146)
  line L138 (-1.705, 3.1949) -> (-1.705, 2.7524)
  line L139 (-1.705, 2.7524) -> (-3.2026, 2.7524)
  spline S168 degree 2 poles (-3.2026, 2.7524) (-3.3841, 2.7524) (-3.6961, 2.7184) (-3.7897, 2.6673) knots 0 0 0 1 2 2 2
  spline S169 degree 2 poles (-3.7897, 2.6673) (-3.889, 2.6134) (-3.9854, 2.4206) (-3.9854, 2.2561) knots 0 0 0 1 2 2 2
  spline S170 degree 2 poles (-3.9854, 2.2561) (-3.9854, 2.0916) (-3.8096, 1.7427) (-3.6678, 1.5754) knots 0 0 0 1 2 2 2
  line L140 (-3.6678, 1.5754) -> (-1.705, 1.5754)
  line L141 (-1.705, 1.5754) -> (-1.705, 1.1329)
  line L142 (-1.705, 1.1329) -> (-4.3314, 1.1329)
  line L143 (-4.3314, 1.1329) -> (-4.3314, 1.5754)
  line L144 (-4.3314, 1.5754) -> (-4.0393, 1.5754)
  spline S171 degree 2 poles (-4.0393, 1.5754) (-4.218, 1.7739) (-4.4052, 2.1568) (-4.4052, 2.3724) knots 0 0 0 1 2 2 2
  spline S172 degree 2 poles (-4.4052, 2.3724) (-4.4052, 2.7581) (-3.8947, 3.1949) (-3.4096, 3.1949) knots 0 0 0 1 2 2 2
  line L145 (-3.4096, 3.1949) -> (-1.705, 3.1949)
  spline S173 degree 2 poles (-1.6455, 4.9562) (-1.6455, 4.3266) (-2.3517, 3.6345) (-3.0041, 3.6345) knots 0 0 0 1 2 2 2
  spline S174 degree 2 poles (-3.0041, 3.6345) (-3.6451, 3.6345) (-4.4052, 4.3067) (-4.4052, 4.8484) knots 0 0 0 1 2 2 2
  spline S175 degree 2 poles (-4.4052, 4.8484) (-4.4052, 5.0924) (-4.2634, 5.4696) (-4.1131, 5.6086) knots 0 0 0 1 2 2 2
  spline S176 degree 2 poles (-4.1131, 5.6086) (-3.9627, 5.7504) (-3.5288, 5.9007) (-3.2139, 5.9007) knots 0 0 0 1 2 2 2
  line L146 (-3.2139, 5.9007) -> (-2.9729, 5.9007)
  line L147 (-2.9729, 5.9007) -> (-2.9729, 4.0826)
  spline S177 degree 2 poles (-2.9729, 4.0826) (-2.5162, 4.0826) (-2.0312, 4.5421) (-2.0312, 4.9506) knots 0 0 0 1 2 2 2
  spline S178 degree 2 poles (-2.0312, 4.9506) (-2.0312, 5.0952) (-2.0964, 5.376) (-2.1475, 5.4895) knots 0 0 0 1 2 2 2
  spline S179 degree 2 poles (-2.1475, 5.4895) (-2.2042, 5.6086) (-2.3035, 5.7731) (-2.3489, 5.827) knots 0 0 0 1 2 2 2
  line L148 (-2.3489, 5.827) -> (-2.3489, 5.8525)
  line L149 (-2.3489, 5.8525) -> (-1.8667, 5.8525)
  spline S180 degree 2 poles (-1.8667, 5.8525) (-1.8355, 5.7759) (-1.7447, 5.5433) (-1.7192, 5.4526) knots 0 0 0 1 2 2 2
  spline S181 degree 2 poles (-1.7192, 5.4526) (-1.6823, 5.3249) (-1.6455, 5.1151) (-1.6455, 4.9562) knots 0 0 0 1 2 2 2
  spline S182 degree 2 poles (-3.3104, 5.4696) (-3.4891, 5.4639) (-3.75, 5.3902) (-3.8379, 5.3193) knots 0 0 0 1 2 2 2
  spline S183 degree 2 poles (-3.8379, 5.3193) (-3.9372, 5.2427) (-4.0421, 5.0016) (-4.0421, 4.8229) knots 0 0 0 1 2 2 2
  spline S184 degree 2 poles (-4.0421, 4.8229) (-4.0421, 4.6471) (-3.9372, 4.4003) (-3.8351, 4.2982) knots 0 0 0 1 2 2 2
  spline S185 degree 2 poles (-3.8351, 4.2982) (-3.7302, 4.1989) (-3.4777, 4.0968) (-3.3104, 4.0826) knots 0 0 0 1 2 2 2
  line L150 (-3.3104, 4.0826) -> (-3.3104, 5.4696)
  line L151 (4.0576, -3.4151) -> (4.0576, -5.1226)
  line L152 (4.0576, -5.1226) -> (3.7003, -5.1226)
  line L153 (3.7003, -5.1226) -> (3.7003, -4.4872)
  line L154 (3.7003, -4.4872) -> (1.3546, -4.4872)
  line L155 (1.3546, -4.4872) -> (1.3546, -5.1226)
  line L156 (1.3546, -5.1226) -> (1.0341, -5.1226)
  spline S186 degree 2 poles (1.0341, -5.1226) (1.0341, -4.7624) (0.8299, -4.422) (0.5463, -4.3993) knots 0 0 0 1 2 2 2
  line L157 (0.5463, -4.3993) -> (0.5463, -4.0363)
  line L158 (0.5463, -4.0363) -> (3.7003, -4.0363)
  line L159 (3.7003, -4.0363) -> (3.7003, -3.4151)
  line L160 (3.7003, -3.4151) -> (4.0576, -3.4151)
  spline S187 degree 2 poles (4.137, -1.7133) (4.137, -1.9743) (3.981, -2.4026) (3.8364, -2.5529) knots 0 0 0 1 2 2 2
  spline S188 degree 2 poles (3.8364, -2.5529) (3.6946, -2.7004) (3.3088, -2.8535) (3.0904, -2.8535) knots 0 0 0 1 2 2 2
  spline S189 degree 2 poles (3.0904, -2.8535) (2.8068, -2.8535) (2.3303, -2.5501) (2.1885, -2.2607) knots 0 0 0 1 2 2 2
  line L161 (2.1885, -2.2607) -> (2.1743, -2.2607)
  spline S190 degree 2 poles (2.1743, -2.2607) (2.024, -2.5189) (1.6666, -2.7684) (1.4, -2.7684) knots 0 0 0 1 2 2 2
  spline S191 degree 2 poles (1.4, -2.7684) (1.0058, -2.7684) (0.4782, -2.1728) (0.4782, -1.7133) knots 0 0 0 1 2 2 2
  spline S192 degree 2 poles (0.4782, -1.7133) (0.4782, -1.2368) (0.9774, -0.6611) (1.3688, -0.6611) knots 0 0 0 1 2 2 2
  spline S193 degree 2 poles (1.3688, -0.6611) (1.6042, -0.6611) (2.0637, -0.9362) (2.1942, -1.1943) knots 0 0 0 1 2 2 2
  line L162 (2.1942, -1.1943) -> (2.2084, -1.1943)
  spline S194 degree 2 poles (2.2084, -1.1943) (2.3502, -0.888) (2.7586, -0.5731) (3.0819, -0.5731) knots 0 0 0 1 2 2 2
  spline S195 degree 2 poles (3.0819, -0.5731) (3.5301, -0.5731) (4.137, -1.2255) (4.137, -1.7133) knots 0 0 0 1 2 2 2
  spline S196 degree 2 poles (3.1273, -1.0553) (2.9118, -1.0553) (2.6565, -1.2255) (2.526, -1.4666) knots 0 0 0 1 2 2 2
  spline S197 degree 2 poles (2.526, -1.4666) (2.4806, -1.546) (2.3757, -1.8126) (2.3076, -1.98) knots 0 0 0 1 2 2 2
  spline S198 degree 2 poles (2.3076, -1.98) (2.4353, -2.1728) (2.8153, -2.3799) (3.0564, -2.3799) knots 0 0 0 1 2 2 2
  spline S199 degree 2 poles (3.0564, -2.3799) (3.3741, -2.3799) (3.7882, -1.997) (3.7882, -1.7077) knots 0 0 0 1 2 2 2
  spline S200 degree 2 poles (3.7882, -1.7077) (3.7882, -1.4127) (3.4336, -1.0553) (3.1273, -1.0553) knots 0 0 0 1 2 2 2
  spline S201 degree 2 poles (1.3745, -1.1206) (1.1391, -1.1206) (0.8242, -1.4354) (0.8242, -1.7162) knots 0 0 0 1 2 2 2
  spline S202 degree 2 poles (0.8242, -1.7162) (0.8242, -1.9714) (1.105, -2.2976) (1.3461, -2.2976) knots 0 0 0 1 2 2 2
  spline S203 degree 2 poles (1.3461, -2.2976) (1.5191, -2.2976) (1.7602, -2.1303) (1.8567, -1.9629) knots 0 0 0 1 2 2 2
  spline S204 degree 2 poles (1.8567, -1.9629) (1.8964, -1.892) (2.0353, -1.5914) (2.0751, -1.4694) knots 0 0 0 1 2 2 2
  spline S205 degree 2 poles (2.0751, -1.4694) (1.9191, -1.2652) (1.5872, -1.1206) (1.3745, -1.1206) knots 0 0 0 1 2 2 2
  line L163 (1.0823, 2.0533) -> (4.0576, 0.5387)
  line L164 (4.0576, 0.5387) -> (4.0576, 0.0395)
  line L165 (4.0576, 0.0395) -> (0.9689, 1.6392)
  line L166 (0.9689, 1.6392) -> (0.9689, -0.1676)
  line L167 (0.9689, -0.1676) -> (0.5576, -0.1676)
  line L168 (0.5576, -0.1676) -> (0.5576, 2.0533)
  line L169 (0.5576, 2.0533) -> (1.0823, 2.0533)
  spline S206 degree 2 poles (4.137, 3.5395) (4.137, 3.2786) (3.981, 2.8503) (3.8364, 2.6999) knots 0 0 0 1 2 2 2
  spline S207 degree 2 poles (3.8364, 2.6999) (3.6946, 2.5525) (3.3088, 2.3993) (3.0904, 2.3993) knots 0 0 0 1 2 2 2
  spline S208 degree 2 poles (3.0904, 2.3993) (2.8068, 2.3993) (2.3303, 2.7028) (2.1885, 2.9921) knots 0 0 0 1 2 2 2
  line L170 (2.1885, 2.9921) -> (2.1743, 2.9921)
  spline S209 degree 2 poles (2.1743, 2.9921) (2.024, 2.734) (1.6666, 2.4844) (1.4, 2.4844) knots 0 0 0 1 2 2 2
  spline S210 degree 2 poles (1.4, 2.4844) (1.0058, 2.4844) (0.4782, 3.08) (0.4782, 3.5395) knots 0 0 0 1 2 2 2
  spline S211 degree 2 poles (0.4782, 3.5395) (0.4782, 4.016) (0.9774, 4.5918) (1.3688, 4.5918) knots 0 0 0 1 2 2 2
  spline S212 degree 2 poles (1.3688, 4.5918) (1.6042, 4.5918) (2.0637, 4.3166) (2.1942, 4.0585) knots 0 0 0 1 2 2 2
  line L171 (2.1942, 4.0585) -> (2.2084, 4.0585)
  spline S213 degree 2 poles (2.2084, 4.0585) (2.3502, 4.3649) (2.7586, 4.6797) (3.0819, 4.6797) knots 0 0 0 1 2 2 2
  spline S214 degree 2 poles (3.0819, 4.6797) (3.5301, 4.6797) (4.137, 4.0273) (4.137, 3.5395) knots 0 0 0 1 2 2 2
  spline S215 degree 2 poles (3.1273, 4.1975) (2.9118, 4.1975) (2.6565, 4.0273) (2.526, 3.7863) knots 0 0 0 1 2 2 2
  spline S216 degree 2 poles (2.526, 3.7863) (2.4806, 3.7068) (2.3757, 3.4402) (2.3076, 3.2729) knots 0 0 0 1 2 2 2
  spline S217 degree 2 poles (2.3076, 3.2729) (2.4353, 3.08) (2.8153, 2.873) (3.0564, 2.873) knots 0 0 0 1 2 2 2
  spline S218 degree 2 poles (3.0564, 2.873) (3.3741, 2.873) (3.7882, 3.2559) (3.7882, 3.5452) knots 0 0 0 1 2 2 2
  spline S219 degree 2 poles (3.7882, 3.5452) (3.7882, 3.8401) (3.4336, 4.1975) (3.1273, 4.1975) knots 0 0 0 1 2 2 2
  spline S220 degree 2 poles (1.3745, 4.1323) (1.1391, 4.1323) (0.8242, 3.8175) (0.8242, 3.5367) knots 0 0 0 1 2 2 2
  spline S221 degree 2 poles (0.8242, 3.5367) (0.8242, 3.2814) (1.105, 2.9552) (1.3461, 2.9552) knots 0 0 0 1 2 2 2
  spline S222 degree 2 poles (1.3461, 2.9552) (1.5191, 2.9552) (1.7602, 3.1226) (1.8567, 3.2899) knots 0 0 0 1 2 2 2
  spline S223 degree 2 poles (1.8567, 3.2899) (1.8964, 3.3608) (2.0353, 3.6615) (2.0751, 3.7834) knots 0 0 0 1 2 2 2
  spline S224 degree 2 poles (2.0751, 3.7834) (1.9191, 3.9876) (1.5872, 4.1323) (1.3745, 4.1323) knots 0 0 0 1 2 2 2
  spline S225 degree 2 poles (8.7453, -13.9548) (9.0063, -13.9548) (9.4062, -14.1534) (9.5367, -14.3179) knots 0 0 0 1 2 2 2
  spline S226 degree 2 poles (9.5367, -14.3179) (9.6898, -14.5164) (9.8203, -14.9674) (9.8203, -15.3248) knots 0 0 0 1 2 2 2
  line L172 (9.8203, -15.3248) -> (9.8203, -16.3288)
  line L173 (9.8203, -16.3288) -> (6.3203, -16.3288)
  line L174 (6.3203, -16.3288) -> (6.3203, -15.4013)
  spline S227 degree 2 poles (6.3203, -15.4013) (6.3203, -15.027) (6.3685, -14.6526) (6.4621, -14.4824) knots 0 0 0 1 2 2 2
  spline S228 degree 2 poles (6.4621, -14.4824) (6.5614, -14.2924) (6.8875, -14.1193) (7.1088, -14.1193) knots 0 0 0 1 2 2 2
  spline S229 degree 2 poles (7.1088, -14.1193) (7.3555, -14.1193) (7.7469, -14.3803) (7.8576, -14.61) knots 0 0 0 1 2 2 2
  line L175 (7.8576, -14.61) -> (7.8746, -14.61)
  spline S230 degree 2 poles (7.8746, -14.61) (7.9597, -14.298) (8.4106, -13.9548) (8.7453, -13.9548) knots 0 0 0 1 2 2 2
  spline S231 degree 2 poles (8.7652, -14.4398) (8.5666, -14.4398) (8.3114, -14.5533) (8.2206, -14.7235) knots 0 0 0 1 2 2 2
  spline S232 degree 2 poles (8.2206, -14.7235) (8.1639, -14.8341) (8.1298, -15.095) (8.1298, -15.3361) knots 0 0 0 1 2 2 2
  line L176 (8.1298, -15.3361) -> (8.1298, -15.8637)
  line L177 (8.1298, -15.8637) -> (9.4232, -15.8637)
  line L178 (9.4232, -15.8637) -> (9.4232, -15.4864)
  spline S233 degree 2 poles (9.4232, -15.4864) (9.4232, -15.1801) (9.3665, -14.8284) (9.2757, -14.6923) knots 0 0 0 1 2 2 2
  spline S234 degree 2 poles (9.2757, -14.6923) (9.1821, -14.5618) (8.9495, -14.4398) (8.7652, -14.4398) knots 0 0 0 1 2 2 2
  spline S235 degree 2 poles (7.174, -14.6043) (7.0492, -14.6043) (6.862, -14.6894) (6.8081, -14.783) knots 0 0 0 1 2 2 2
  spline S236 degree 2 poles (6.8081, -14.783) (6.7457, -14.8965) (6.7174, -15.1716) (6.7174, -15.4184) knots 0 0 0 1 2 2 2
  line L179 (6.7174, -15.4184) -> (6.7174, -15.8637)
  line L180 (6.7174, -15.8637) -> (7.7413, -15.8637)
  line L181 (7.7413, -15.8637) -> (7.7413, -15.3361)
  spline S237 degree 2 poles (7.7413, -15.3361) (7.7413, -15.1177) (7.6959, -14.9107) (7.625, -14.8001) knots 0 0 0 1 2 2 2
  spline S238 degree 2 poles (7.625, -14.8001) (7.5569, -14.6923) (7.3385, -14.6043) (7.174, -14.6043) knots 0 0 0 1 2 2 2
  line L182 (7.1939, -11.4646) -> (10.7875, -12.877)
  line L183 (10.7875, -12.877) -> (10.7875, -13.3507)
  line L184 (10.7875, -13.3507) -> (9.6927, -12.8799)
  line L185 (9.6927, -12.8799) -> (7.1939, -13.8329)
  line L186 (7.1939, -13.8329) -> (7.1939, -13.3564)
  line L187 (7.1939, -13.3564) -> (9.1396, -12.6388)
  line L188 (9.1396, -12.6388) -> (7.1939, -11.924)
  line L189 (7.1939, -11.924) -> (7.1939, -11.4646)
  line L190 (9.8203, -10.3187) -> (9.8203, -10.8803)
  line L191 (9.8203, -10.8803) -> (9.1509, -10.8803)
  line L192 (9.1509, -10.8803) -> (9.1509, -10.3187)
  line L193 (9.1509, -10.3187) -> (9.8203, -10.3187)
  line L194 (7.8632, -10.3187) -> (7.8632, -10.8803)
  line L195 (7.8632, -10.8803) -> (7.1939, -10.8803)
  line L196 (7.1939, -10.8803) -> (7.1939, -10.3187)
  line L197 (7.1939, -10.3187) -> (7.8632, -10.3187)
  line L198 (9.8203, -8.268) -> (6.3203, -7.0881)
  line L199 (6.3203, -7.0881) -> (6.3203, -6.5152)
  line L200 (6.3203, -6.5152) -> (9.8203, -5.3353)
  line L201 (9.8203, -5.3353) -> (9.8203, -5.826)
  line L202 (9.8203, -5.826) -> (8.8418, -6.1437)
  line L203 (8.8418, -6.1437) -> (8.8418, -7.4796)
  line L204 (8.8418, -7.4796) -> (9.8203, -7.7972)
  line L205 (9.8203, -7.7972) -> (9.8203, -8.268)
  line L206 (8.4447, -6.2713) -> (6.7968, -6.813)
  line L207 (6.7968, -6.813) -> (8.4447, -7.3519)
  line L208 (8.4447, -7.3519) -> (8.4447, -6.2713)
  line L209 (9.8203, -2.0594) -> (8.3, -2.0594)
  spline S239 degree 2 poles (8.3, -2.0594) (8.1185, -2.0594) (7.8093, -2.0877) (7.7243, -2.1331) knots 0 0 0 1 2 2 2
  spline S240 degree 2 poles (7.7243, -2.1331) (7.6307, -2.1785) (7.5399, -2.3515) (7.5399, -2.5018) knots 0 0 0 1 2 2 2
  spline S241 degree 2 poles (7.5399, -2.5018) (7.5399, -2.638) (7.7072, -2.95) (7.8661, -3.1145) knots 0 0 0 1 2 2 2
  spline S242 degree 2 poles (7.8661, -3.1145) (7.9058, -3.1116) (8.0164, -3.106) (8.0901, -3.106) knots 0 0 0 1 2 2 2
  line L210 (8.0901, -3.106) -> (9.8203, -3.106)
  line L211 (9.8203, -3.106) -> (9.8203, -3.5484)
  line L212 (9.8203, -3.5484) -> (8.3, -3.5484)
  spline S243 degree 2 poles (8.3, -3.5484) (8.1185, -3.5484) (7.8093, -3.5768) (7.7243, -3.6222) knots 0 0 0 1 2 2 2
  spline S244 degree 2 poles (7.7243, -3.6222) (7.6307, -3.6676) (7.5399, -3.8406) (7.5399, -3.9909) knots 0 0 0 1 2 2 2
  spline S245 degree 2 poles (7.5399, -3.9909) (7.5399, -4.1327) (7.7186, -4.4475) (7.8576, -4.595) knots 0 0 0 1 2 2 2
  line L213 (7.8576, -4.595) -> (9.8203, -4.595)
  line L214 (9.8203, -4.595) -> (9.8203, -5.0375)
  line L215 (9.8203, -5.0375) -> (7.1939, -5.0375)
  line L216 (7.1939, -5.0375) -> (7.1939, -4.595)
  line L217 (7.1939, -4.595) -> (7.4832, -4.595)
  spline S246 degree 2 poles (7.4832, -4.595) (7.3102, -4.422) (7.1201, -4.0817) (7.1201, -3.8774) knots 0 0 0 1 2 2 2
  spline S247 degree 2 poles (7.1201, -3.8774) (7.1201, -3.6449) (7.3328, -3.2847) (7.5739, -3.1911) knots 0 0 0 1 2 2 2
  spline S248 degree 2 poles (7.5739, -3.1911) (7.3499, -2.9897) (7.1201, -2.6096) (7.1201, -2.3884) knots 0 0 0 1 2 2 2
  spline S249 degree 2 poles (7.1201, -2.3884) (7.1201, -2.2182) (7.2251, -1.9402) (7.3442, -1.8381) knots 0 0 0 1 2 2 2
  spline S250 degree 2 poles (7.3442, -1.8381) (7.4633, -1.7332) (7.8207, -1.6169) (8.0901, -1.6169) knots 0 0 0 1 2 2 2
  line L218 (8.0901, -1.6169) -> (9.8203, -1.6169)
  line L219 (9.8203, -1.6169) -> (9.8203, -2.0594)
  spline S251 degree 2 poles (8.5071, 1.1627) (9.1708, 1.1627) (9.894, 0.5245) (9.894, -0.0087) knots 0 0 0 1 2 2 2
  spline S252 degree 2 poles (9.894, -0.0087) (9.894, -0.5561) (9.1481, -1.183) (8.5071, -1.183) knots 0 0 0 1 2 2 2
  spline S253 degree 2 poles (8.5071, -1.183) (7.8491, -1.183) (7.1201, -0.5363) (7.1201, -0.0087) knots 0 0 0 1 2 2 2
  spline S254 degree 2 poles (7.1201, -0.0087) (7.1201, 0.5245) (7.8462, 1.1627) (8.5071, 1.1627) knots 0 0 0 1 2 2 2
  spline S255 degree 2 poles (8.5071, 0.706) (7.9965, 0.706) (7.5002, 0.3345) (7.5002, -0.0087) knots 0 0 0 1 2 2 2
  spline S256 degree 2 poles (7.5002, -0.0087) (7.5002, -0.3519) (7.9965, -0.7263) (8.5071, -0.7263) knots 0 0 0 1 2 2 2
  spline S257 degree 2 poles (8.5071, -0.7263) (9.0034, -0.7263) (9.514, -0.3519) (9.514, -0.0087) knots 0 0 0 1 2 2 2
  spline S258 degree 2 poles (9.514, -0.0087) (9.514, 0.3316) (9.0119, 0.706) (8.5071, 0.706) knots 0 0 0 1 2 2 2
  line L220 (9.8203, 2.0675) -> (9.8203, 1.625)
  line L221 (9.8203, 1.625) -> (6.1643, 1.625)
  line L222 (6.1643, 1.625) -> (6.1643, 2.0675)
  line L223 (6.1643, 2.0675) -> (9.8203, 2.0675)
  spline S259 degree 2 poles (8.7453, 6.6282) (9.0063, 6.6282) (9.4062, 6.4297) (9.5367, 6.2652) knots 0 0 0 1 2 2 2
  spline S260 degree 2 poles (9.5367, 6.2652) (9.6898, 6.0666) (9.8203, 5.6157) (9.8203, 5.2583) knots 0 0 0 1 2 2 2
  line L224 (9.8203, 5.2583) -> (9.8203, 4.2542)
  line L225 (9.8203, 4.2542) -> (6.3203, 4.2542)
  line L226 (6.3203, 4.2542) -> (6.3203, 5.1817)
  spline S261 degree 2 poles (6.3203, 5.1817) (6.3203, 5.5561) (6.3685, 5.9305) (6.4621, 6.1007) knots 0 0 0 1 2 2 2
  spline S262 degree 2 poles (6.4621, 6.1007) (6.5614, 6.2907) (6.8875, 6.4637) (7.1088, 6.4637) knots 0 0 0 1 2 2 2
  spline S263 degree 2 poles (7.1088, 6.4637) (7.3555, 6.4637) (7.7469, 6.2028) (7.8576, 5.973) knots 0 0 0 1 2 2 2
  line L227 (7.8576, 5.973) -> (7.8746, 5.973)
  spline S264 degree 2 poles (7.8746, 5.973) (7.9597, 6.285) (8.4106, 6.6282) (8.7453, 6.6282) knots 0 0 0 1 2 2 2
  spline S265 degree 2 poles (8.7652, 6.1432) (8.5666, 6.1432) (8.3114, 6.0298) (8.2206, 5.8596) knots 0 0 0 1 2 2 2
  spline S266 degree 2 poles (8.2206, 5.8596) (8.1639, 5.749) (8.1298, 5.488) (8.1298, 5.2469) knots 0 0 0 1 2 2 2
  line L228 (8.1298, 5.2469) -> (8.1298, 4.7194)
  line L229 (8.1298, 4.7194) -> (9.4232, 4.7194)
  line L230 (9.4232, 4.7194) -> (9.4232, 5.0966)
  spline S267 degree 2 poles (9.4232, 5.0966) (9.4232, 5.4029) (9.3665, 5.7546) (9.2757, 5.8908) knots 0 0 0 1 2 2 2
  spline S268 degree 2 poles (9.2757, 5.8908) (9.1821, 6.0213) (8.9495, 6.1432) (8.7652, 6.1432) knots 0 0 0 1 2 2 2
  spline S269 degree 2 poles (7.174, 5.9787) (7.0492, 5.9787) (6.862, 5.8936) (6.8081, 5.8) knots 0 0 0 1 2 2 2
  spline S270 degree 2 poles (6.8081, 5.8) (6.7457, 5.6866) (6.7174, 5.4115) (6.7174, 5.1647) knots 0 0 0 1 2 2 2
  line L231 (6.7174, 5.1647) -> (6.7174, 4.7194)
  line L232 (6.7174, 4.7194) -> (7.7413, 4.7194)
  line L233 (7.7413, 4.7194) -> (7.7413, 5.2469)
  spline S271 degree 2 poles (7.7413, 5.2469) (7.7413, 5.4653) (7.6959, 5.6724) (7.625, 5.783) knots 0 0 0 1 2 2 2
  spline S272 degree 2 poles (7.625, 5.783) (7.5569, 5.8908) (7.3385, 5.9787) (7.174, 5.9787) knots 0 0 0 1 2 2 2
  line L234 (9.8203, 9.0986) -> (9.8203, 8.6562)
  line L235 (9.8203, 8.6562) -> (9.531, 8.6562)
  spline S273 degree 2 poles (9.531, 8.6562) (9.7097, 8.452) (9.894, 8.0861) (9.894, 7.8592) knots 0 0 0 1 2 2 2
  spline S274 degree 2 poles (9.894, 7.8592) (9.894, 7.689) (9.7806, 7.3855) (9.6586, 7.2749) knots 0 0 0 1 2 2 2
  spline S275 degree 2 poles (9.6586, 7.2749) (9.5367, 7.1615) (9.1651, 7.0367) (8.8985, 7.0367) knots 0 0 0 1 2 2 2
  line L236 (8.8985, 7.0367) -> (7.1939, 7.0367)
  line L237 (7.1939, 7.0367) -> (7.1939, 7.4791)
  line L238 (7.1939, 7.4791) -> (8.6914, 7.4791)
  spline S276 degree 2 poles (8.6914, 7.4791) (8.9013, 7.4791) (9.1764, 7.5103) (9.2786, 7.5642) knots 0 0 0 1 2 2 2
  spline S277 degree 2 poles (9.2786, 7.5642) (9.3807, 7.6181) (9.4743, 7.8025) (9.4743, 7.9755) knots 0 0 0 1 2 2 2
  spline S278 degree 2 poles (9.4743, 7.9755) (9.4743, 8.1371) (9.2899, 8.503) (9.1566, 8.6562) knots 0 0 0 1 2 2 2
  line L239 (9.1566, 8.6562) -> (7.1939, 8.6562)
  line L240 (7.1939, 8.6562) -> (7.1939, 9.0986)
  line L241 (7.1939, 9.0986) -> (9.8203, 9.0986)
  line L242 (9.8203, 10.1906) -> (9.8203, 9.7482)
  line L243 (9.8203, 9.7482) -> (6.1643, 9.7482)
  line L244 (6.1643, 9.7482) -> (6.1643, 10.1906)
  line L245 (6.1643, 10.1906) -> (9.8203, 10.1906)
  line L246 (9.8203, 11.2911) -> (9.8203, 10.8486)
  line L247 (9.8203, 10.8486) -> (6.1643, 10.8486)
  line L248 (6.1643, 10.8486) -> (6.1643, 11.2911)
  line L249 (6.1643, 11.2911) -> (9.8203, 11.2911)
  spline S279 degree 2 poles (9.5423, 13.4042) (9.582, 13.3503) (9.7239, 13.1687) (9.7664, 13.0837) knots 0 0 0 1 2 2 2
  spline S280 degree 2 poles (9.7664, 13.0837) (9.8288, 12.9674) (9.894, 12.749) (9.894, 12.5504) knots 0 0 0 1 2 2 2
  spline S281 degree 2 poles (9.894, 12.5504) (9.894, 12.3888) (9.7721, 12.0966) (9.6615, 11.986) knots 0 0 0 1 2 2 2
  spline S282 degree 2 poles (9.6615, 11.986) (9.5537, 11.8811) (9.236, 11.7534) (9.0602, 11.7534) knots 0 0 0 1 2 2 2
  spline S283 degree 2 poles (9.0602, 11.7534) (8.7879, 11.7534) (8.4021, 11.9832) (8.2915, 12.2328) knots 0 0 0 1 2 2 2
  spline S284 degree 2 poles (8.2915, 12.2328) (8.1894, 12.454) (8.1128, 13.0553) (8.093, 13.4042) knots 0 0 0 1 2 2 2
  line L250 (8.093, 13.4042) -> (8.0079, 13.4042)
  spline S285 degree 2 poles (8.0079, 13.4042) (7.8547, 13.4042) (7.6647, 13.3106) (7.6108, 13.2255) knots 0 0 0 1 2 2 2
  spline S286 degree 2 poles (7.6108, 13.2255) (7.5569, 13.1404) (7.5229, 12.8965) (7.5229, 12.766) knots 0 0 0 1 2 2 2
  spline S287 degree 2 poles (7.5229, 12.766) (7.5229, 12.6128) (7.6136, 12.1987) (7.7016, 11.9917) knots 0 0 0 1 2 2 2
  line L251 (7.7016, 11.9917) -> (7.7016, 11.9662)
  line L252 (7.7016, 11.9662) -> (7.2506, 11.9662)
  spline S288 degree 2 poles (7.2506, 11.9662) (7.2166, 12.0881) (7.1315, 12.5448) (7.1315, 12.7688) knots 0 0 0 1 2 2 2
  spline S289 degree 2 poles (7.1315, 12.7688) (7.1315, 13.0411) (7.2166, 13.4127) (7.3272, 13.5602) knots 0 0 0 1 2 2 2
  spline S290 degree 2 poles (7.3272, 13.5602) (7.435, 13.7048) (7.7781, 13.8466) (8.0249, 13.8466) knots 0 0 0 1 2 2 2
  line L253 (8.0249, 13.8466) -> (9.8203, 13.8466)
  line L254 (9.8203, 13.8466) -> (9.8203, 13.4042)